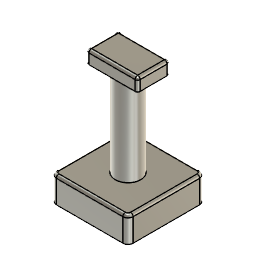
Hanging Hook (Autodesk Fusion 360 design; units mm, degrees)
Autodesk Fusion 360 part; units mm, degrees
sketch "Sketch1" plane through (0, 0, 0) normal (0, 0, 1) x (1, 0, 0)
  circle A0 centre (0, 0) radius 10
  line L0 (18, 12.5) -> (-18, 12.5)
  line L1 (-20, 10.5) -> (-20, -10.5)
  line L2 (-18, -12.5) -> (18, -12.5)
  line L3 (20, -10.5) -> (20, 10.5)
  line L4 (20, 12.5) -> (-20, -12.5) construction
  line L5 (-20, 12.5) -> (20, -12.5) construction
  arc A1 (20, 10.5) -> (18, 12.5) centre (18, 10.5) ccw
  arc A2 (18, -12.5) -> (20, -10.5) centre (18, -10.5) ccw
  arc A3 (-20, -10.5) -> (-18, -12.5) centre (-18, -10.5) ccw
  arc A4 (-18, 12.5) -> (-20, 10.5) centre (-18, 10.5) ccw
  dimension "d1" = 20
  dimension "d2" = 40
  dimension "d3" = 25
  dimension "d4" = 2
  dimension "d5" = 2
  dimension "d6" = 2
  constraint coincident A0.centre origin
  constraint horizontal L0
  constraint perpendicular L0 L1
  constraint parallel L0 L2
  constraint parallel L1 L3
  constraint coincident L4 A0.centre
  constraint coincident L5 A0.centre
  constraint coincident L4.start L3
  constraint coincident L4.start L0
  constraint tangent L3 A1
  constraint tangent L0 A1
  constraint coincident L5.end L3
  constraint coincident L5.end L2
  constraint tangent L3 A2
  constraint tangent L2 A2
  constraint equal A1 A2
  constraint coincident L4.end L1
  constraint coincident L4.end L2
  constraint tangent L1 A3
  constraint tangent L2 A3
  constraint coincident L5.start L0
  constraint coincident L5.start L1
  constraint tangent L0 A4
  constraint tangent L1 A4
  measures "d1" diameter of A0
  measures "d2" distance of L4.end L5.end
  measures "d3" distance of L5.start L4.end
  measures "d4" radius of A1
  measures "d5" radius of A3
  measures "d6" radius of A4
extrude "Extrude1" add sketch "Sketch1" along normal blind 10
extrude "Extrude2" add sketch "Sketch1" along normal blind 80 contours A0
sketch "Sketch2" plane through (0, 0, 80) normal (0, 0, 1) x (-1, 0, 0)
  circle A0 centre (0, 0) radius 10
  line L0 (-26, -30) -> (26, -30)
  line L1 (30, -26) -> (30, 26)
  line L2 (26, 30) -> (-26, 30)
  line L3 (-30, 26) -> (-30, -26)
  line L4 (-30, -30) -> (30, 30) construction
  line L5 (30, -30) -> (-30, 30) construction
  arc A1 (-30, -26) -> (-26, -30) centre (-26, -26) ccw
  arc A2 (-26, 30) -> (-30, 26) centre (-26, 26) ccw
  arc A3 (30, 26) -> (26, 30) centre (26, 26) ccw
  arc A4 (26, -30) -> (30, -26) centre (26, -26) ccw
  dimension "d11" = 60
  dimension "d12" = 60
  dimension "d13" = 4
  dimension "d14" = 4
  dimension "d15" = 4
  dimension "d16" = 4
  constraint horizontal L0
  constraint perpendicular L0 L1
  constraint parallel L0 L2
  constraint parallel L1 L3
  constraint coincident L4 A0.centre
  constraint coincident L5 A0.centre
  constraint coincident A0.centre origin
  constraint coincident L4.start L0
  constraint coincident L4.start L3
  constraint tangent L0 A1
  constraint tangent L3 A1
  constraint coincident L5.end L3
  constraint coincident L5.end L2
  constraint tangent L3 A2
  constraint tangent L2 A2
  constraint coincident L4.end L1
  constraint coincident L4.end L2
  constraint tangent L1 A3
  constraint tangent L2 A3
  constraint coincident L5.start L1
  constraint coincident L5.start L0
  constraint tangent L1 A4
  constraint tangent L0 A4
  measures "d11" distance of L4.end L5.end
  measures "d12" distance of L5.start L4.end
  measures "d13" radius of A1
  measures "d14" radius of A2
  measures "d15" radius of A3
  measures "d16" radius of A4
extrude "Extrude3" add sketch "Sketch2" along normal blind 20 contours A0 | L0 L1 L2 L3 A1 A2 A3 A4
move_body "Move1" bodies 1 to x (-1, 0, 0) y (0, 1, 0) z (0, 0, -1) at (0, 0, 100)
fillet "Fillet1" radius 2 8 edges at (-20, 0, 100) (-19.4142, 11.9142, 100) (0, 12.5, 100) (19.4142, 11.9142, 100) (20, 0, 100) (19.4142, -11.9142, 100) (0, -12.5, 100) (-19.4142, -11.9142, 100)
fillet "Fillet2" radius 2 8 edges at (30, 0, 20) (28.8284, -28.8284, 20) (0, -30, 20) (-28.8284, -28.8284, 20) (-30, 0, 20) (-28.8284, 28.8284, 20) (0, 30, 20) (28.8284, 28.8284, 20)
